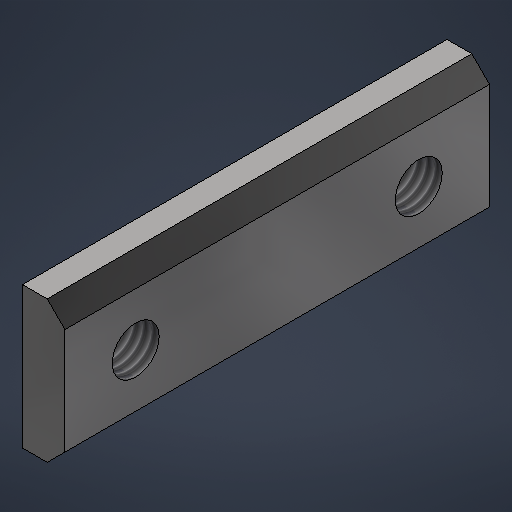
# Autodesk Inventor part: NUT, MK 2/40, M8
Saved by Autodesk Inventor 2026.1 (Build 301233020, 233B)
## iProperties
Manager: 100-30423
Category: _
Part Number: NUT, MK 2/40, M8
Material: Steel, Alloy
Document SubType Name: Modeling
Created: 2007-10-19
Designer: dan.paquette
Manufacturer: Standard
Standards Organization: Custom
Checked By: 1DN66
User Status: Work In Process
Description: NUT, MK 2/40, M8
Engr Approved By: R
Mfg Approved By: Dan.Paquette
Density: 7.73 g/cm^3
Appearance: Semi-Polished
Mass: 49.5384 g
Surface Area: 32.8355 cm^2
Volume: 6.40859 cm^3
Control State: 0
Master: False
Checked Out: False
Shininess: 64.0
Angle Display Precision: 2
Document Length Units: 11269
Document Angle Units: 11279
Document Time Units: 11290
Document Mass Units: 11286
Document Length Units Precision: 3
Document Angle Units Precision: 2
Translation Standard: STEP AP214DIS
File Name: //partserver001.servicenet/client_exchange/iodir/jobs/output/wkb8294367_no0/STEP/34_01_0019_2_14a.stp
Postprocessor: Build: 081d, Release: 8 SP1 - Date: Tue 01/26/2004
Sent Units: MILLIMETERS
Uncertainty: 1.0000000000000002e-06
CN_SERVICEABLE: _
FIRST_DESCRIPTION: NUT, MK 2/40, M8
PTC_WM_ITERATION: 4
PTC_WM_ORGANIZATION_ID: CLWC
PTC_WM_LIFECYCLE: CLWC_CAD_LC
CN_MASS: 0.05021108161748321
CL_runCount: 1
FinishProperty: ToBeSet
SECOND_DESCRIPTION: _
THIRD_DESCRIPTION: _
Density: 0.0
Volumn: 0.0
Area: 0.0
PropertySet Name: Model Information
Title: plate nut,MK,34_01_0019_1DN66.ipt
Subject: 34.01.0019
Author: -
Keywords: MK
Revision Number: 1
Autodesk Inventor part; units mm, degrees
ref_plane "YZ Plane" through (0, 0, 0) normal (1, 0, 0) x (0, 1, 0)
ref_plane "XZ Plane" through (0, 0, 0) normal (0, 1, 0) x (-1, 0, 0)
ref_plane "XY Plane" through (0, 0, 0) normal (0, 0, 1) x (1, 0, 0)
sketch "Sketch1" plane through (0, 0, 0) normal (0, 0, 1) x (1, 0, 0)
  line L0 (0, -10) -> (3.5, -10)
  line L1 (0, 10) -> (0, -10)
  line L2 (3.5, 10) -> (0, 10)
  line L3 (6, 7.5) -> (3.5, 10)
  line L4 (6, -7.5) -> (6, 7.5)
  line L5 (3.5, -10) -> (6, -7.5)
  line L6 (-1.2, 0) -> (7.2, 0) construction
  line L7 (0, -14) -> (0, 14) construction
  dimension "d0" = 20
  dimension "d1" = 15
  dimension "d2" = 45
  dimension "d3" = 6
  constraints: 12 end point, 1 collinear, 1 perpendicular, 2 other
  measures "d0" distance of L1.start L0.start
  measures "d1" distance of L4.start L3.start
  measures "d2" angle of L0 L5
  measures "d3" distance between parallel lines of L1 L4
extrude "Extrusion1" add sketch "Sketch1" along normal mid plane 60
sketch "Sketch2" plane through (0, -10, 30) normal (-1, 0, 0) x (0, 0, 1)
  line L0 (-72, 10) -> (12, 10) construction
  line L1 (-30, -4) -> (-30, 24) construction
  point P0 (-30, 10)
  point P1 (-50, 10)
  point P2 (-10, 10)
  dimension "d6" = 40
  constraints: 2 point on line, 1 symmetric about line
  measures "d6" distance of point (-10, 10) point (-50, 10)
hole "Hole1" at (0, 0, -20) at (0, 0, 20) direction (1, 0, 0) diameter 6.647 end through all thread size "M8x1.25" class "6H" standard "ANSI Metric M Profile"
body "Solid2"
